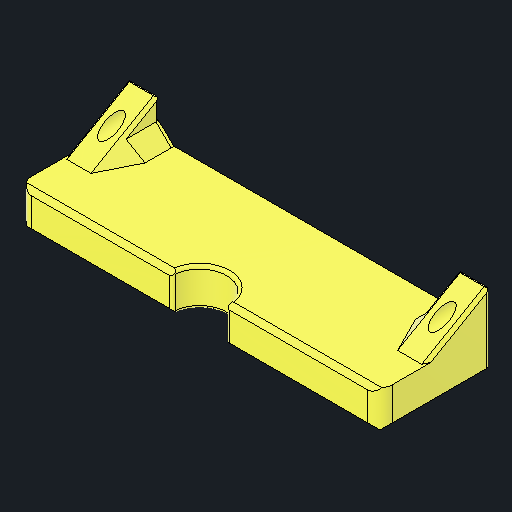
# Autodesk Inventor part: ProbeRest_smaller_variant
Saved by Autodesk Inventor 2026 (Build 300175050, 175E)
## iProperties
Created: 2023-08-17
Part Number: ProbeRest_smaller_variant
Material: Generic
Document SubType Name: Modeling
Designer: kuzmin
Density: 1 g/cm^3
Appearance: Smooth - Yellow
Author: kuzmin
Autodesk Inventor part; units mm, degrees
ref_plane "YZ Plane" through (0, 0, 0) normal (1, 0, 0) x (0, 1, 0)
ref_plane "XZ Plane" through (0, 0, 0) normal (0, 1, 0) x (-1, 0, 0)
sketch "Sketch3" plane through (0, 0, 0) normal (0, 0, 1) x (1, 0, 0)
  arc A0 (18, 0) -> (-18, 0) centre (0, 0) ccw
  line L0 (-18, 0) -> (-120, 0)
  line L1 (18, 0) -> (120, 0)
  line L2 (-120, 0) -> (-120, 73)
  line L3 (-120, 73) -> (120, 73)
  line L4 (120, 73) -> (120, 0)
  point P0 (0, 18)
  dimension "d11" = 36
  dimension "d43" = 240
  dimension "d44" = 73
  constraints: 10 end point, 3 point on circle, 2 collinear, 2 perpendicular, 2 point on line, 1 centre point, 1 coincident, 1 horizontal, 1 vertical
  measures "d11" diameter of A0
  measures "d43" distance of L2.end L3.end
  measures "d44" distance of L0.end L2.end
extrude "Extrusion3" add sketch "Sketch3" along normal blind 25
sketch "Sketch7" plane through (120, 0, 0) normal (1, 0, 0) x (0, 0, -1)
  line L0 (-25, 0) -> (-25, 73) projected
  line L1 (-25, 29.6987) -> (-25, 73)
  line L2 (-25, 73) -> (-50, 73)
  line L3 (-50, 73) -> (-25, 29.6987)
  point P0 (0, 0)
  dimension "d45" = 25
  dimension "d46" = 30
  constraints: 6 end point, 1 collinear, 1 perpendicular, 1 point on line
  measures "d45" distance of L0.end L2.end
  measures "d46" angle of L0 L3
extrude "Extrusion7" add sketch "Sketch7" against normal blind 20
mirror "Mirror1" about plane through (0, 0, 0) normal (1, 0, 0) of "Extrusion7"
sketch "Sketch8" plane through (-120, 73, 0) normal (0, 1, 0) x (1, 0, 0)
  line L0 (20, -50) -> (20, -25) projected
  line L1 (0, 0) -> (0, -50) projected
  line L2 (0, -50) -> (20, -50) projected
  line L3 (12, -25) -> (8, -25)
  line L4 (8, -25) -> (8, -5)
  line L5 (8, -5) -> (12, -5)
  line L6 (12, -5) -> (12, -25)
  line L7 (220, -25) -> (20, -25) projected
  line L8 (240, 0) -> (0, 0) projected
  point P0 (120, 0)
  point P1 (10, -25)
  point P2 (10, -50)
  dimension "d49" = 4
  dimension "d50" = 5
  constraints: 8 end point, 2 midpoint, 2 parallel, 1 horizontal, 1 perpendicular, 1 point on line, 1 vertical alignment
  measures "d49" distance of L3.start L3.end
  measures "d50" distance between parallel lines of L8 L5
extrude "Extrusion8" add sketch "Sketch8" along normal blind 2
chamfer "Chamfer5" distance 2 angle 45 2 edges at (-110, 75, 5) (-110, 75, 25)
sketch "Sketch9" plane through (-120, 73, 0) normal (0, 1, 0) x (1, 0, 0)
  circle A0 centre (10, -37.5) radius 2.9
  line L0 (0, -50) -> (20, -50) projected
  line L1 (20, -50) -> (20, -25) projected
  point P0 (120, 0)
  point P1 (10, -50)
  point P2 (20, -37.5)
  dimension "d56" = 5.8
  constraints: 2 midpoint, 1 centre point, 1 horizontal alignment, 1 vertical alignment
  measures "d56" diameter of A0
extrude "Extrusion9" cut sketch "Sketch9" against normal through all
ref_plane "Work Plane1" through (-120, 68, 0) normal (0, 1, 0) x (1, 0, 0)
sketch "Sketch10" plane through (-120, 68, 0) normal (0, 1, 0) x (1, 0, 0)
  circle A0 centre (10, -37.5) radius 2.9 projected
  circle A1 centre (10, -37.5) radius 4.65
  point P0 (120, 0)
  dimension "d60" = 9.3
  constraints: 1 centre point, 1 coincident
  measures "d60" diameter of A1
extrude "Extrusion10" cut sketch "Sketch10" against normal through all contours A0 | A1
mirror "Mirror2" about plane through (0, 0, 0) normal (1, 0, 0) of "Extrusion8", "Extrusion10", "Extrusion9"
chamfer "Chamfer6" distance 3 angle 45 7 edges at (0, 73, 0) (120, 36.5, 0) (69, 0, 0) (-69, 0, 0) (-120, 36.5, 0) (-69, 0, 25) (69, 0, 25)
chamfer "Chamfer7" distance 2 angle 45 2 edges at (110, 75, 5) (110, 75, 25)
chamfer "Chamfer8" distance 2 angle 45 6 edges at (100, 51.3494, 37.5) (120, 51.3494, 37.5) (-100, 51.3494, 37.5) (-120, 51.3494, 37.5) (-110, 73, 50) (110, 73, 50)
fillet "Fillet4" radius 2 2 edges at (0, 18, 25) (0, 18, 0)
fillet "Fillet5" radius 2 2 edges at (-18, 0, 12.5) (18, 0, 12.5)
fillet "Fillet6" radius 8 2 edges at (120, 0, 12.5) (-120, 0, 12.5)
fillet "Fillet7" radius 2 4 edges at (120, 73, 25.3453) (100, 73, 36.3453) (-100, 73, 36.3453) (-120, 73, 25.3453)
chamfer "Chamfer13" distance 10 angle 45 4 edges at (100, 52.3494, 25) (100.5858, 72.4142, 25) (-100, 52.3494, 25) (-100.5858, 72.4142, 25)
sketch "Sketch19" plane through (-117, 0, 3) normal (0, -1, 0) x (1, 0, 0)
  line L0 (207, 9.5) -> (27, 9.5) construction
  line L1 (0, 0) -> (0, 19) projected
  point P0 (117, -3)
  point P1 (117, 9.5)
  point P2 (0, 9.5)
  dimension "d171" = 180
  constraints: 2 coincident, 2 end point, 2 midpoint, 1 horizontal, 1 horizontal alignment, 1 vertical alignment
  measures "d171" distance of L0.start L0.end
sketch "Sketch18" plane through (-120, 3, 3) normal (-1, 0, 0) x (0, 0, 1)
  line L0 (22, 0) -> (22, 17) construction
  line L1 (22, 30.6987) -> (22, 26.6987) construction
  line L2 (22, 26.6987) -> (-3, 26.6987)
  line L3 (-3, 0) -> (-3, 67) projected
  point P0 (-3, -3)
  constraints: 2 end point, 1 horizontal, 1 point on line
body "Solid2"
body "Solid3"
body "Solid4"
